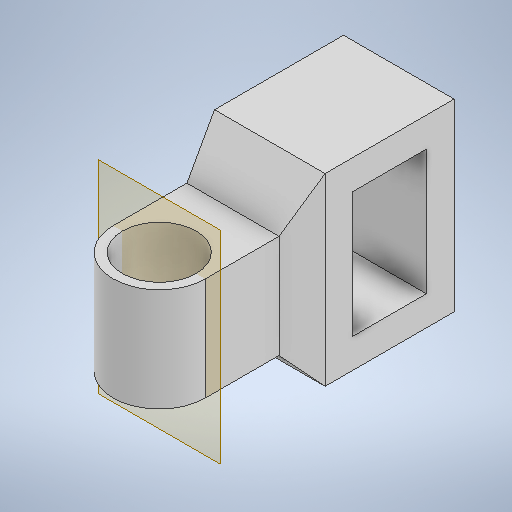
# Autodesk Inventor part: Part5
Saved by Autodesk Inventor 2025.2 (Build 292293000, 293)
## iProperties
Created: 2025-04-11
Part Number: Part5
Material: Generic
Document SubType Name: Sheet Metal
Designer: ziyuz
Density: 1 g/cm^3
Sheet Metal Rule: Default_mm
Appearance: Default
Author: ziyuz
Autodesk Inventor part; units mm, degrees
ref_plane "YZ Plane" through (0, 0, 0) normal (1, 0, 0) x (0, 1, 0)
ref_plane "XZ Plane" through (0, 0, 0) normal (0, 1, 0) x (-1, 0, 0)
sketch "Sketch1" plane through (0, 0, 0) normal (0, 1, 0) x (-1, 0, 0)
  circle A0 centre (0, 0) radius 10
  circle A1 centre (0, 0) radius 12.5
  dimension "d0" = 20
  dimension "d1" = 25
  constraints: 2 centre point, 2 coincident
  measures "d0" diameter of A0
  measures "d1" diameter of A1
extrude "Extrusion1" add sketch "Sketch1" along normal blind 28
sketch "Sketch2" plane through (0, 0, 0) normal (0, 0, 1) x (1, 0, 0)
  line L0 (12.5, 0) -> (-12.5, 0) projected
  line L1 (12.5, 28) -> (-12.5, 28) projected
  line L2 (-12.5, 0) -> (12.5, 0)
  line L3 (12.5, 0) -> (12.5, 28)
  line L4 (12.5, 28) -> (-12.5, 28)
  line L5 (-12.5, 28) -> (-12.5, 0)
  point P0 (0, 0)
  constraints: 8 end point, 2 parallel, 1 horizontal, 1 perpendicular
extrude "Extrusion2" add sketch "Sketch2" against normal blind 20
sketch "Sketch3" plane through (0, 28, 0) normal (0, 1, 0) x (1, 0, 0)
  circle A0 centre (0, 0) radius 10
  constraints: 1 centre point, 1 coincident
extrude "Extrusion3" cut sketch "Sketch3" against normal blind 50
ref_plane "Work Plane1" through (0, 0, -30) normal (0, 0, -1) x (-1, 0, 0)
sketch "Sketch4" plane through (0, 0, -30) normal (0, 0, -1) x (-1, 0, 0)
  line L0 (0, 0) -> (0, 28)
  line L1 (12.5, 28) -> (-12.5, 28) projected
  line L2 (-15, 30) -> (15, 30)
  line L3 (15, 30) -> (15, -2)
  line L4 (15, -2) -> (-15, -2)
  line L5 (-15, -2) -> (-15, 30)
  line L6 (-15, 30) -> (15, -2) construction
  line L7 (15, 30) -> (-15, -2) construction
  point P0 (0, 14)
  dimension "d9" = 30
  dimension "d10" = 32
  constraints: 14 end point, 4 midpoint, 2 parallel, 1 horizontal, 1 perpendicular
  measures "d9" distance of L3.end L4.end
  measures "d10" distance of L2.end L3.end
extrude "Extrusion4" add sketch "Sketch4" along normal blind 15
sketch "Sketch5" plane through (0, 0, -45) normal (0, 0, -1) x (-1, 0, 0)
  line L0 (15, 30) -> (-15, 30) projected
  line L1 (0, 30) -> (0, -2)
  line L2 (-15, -2) -> (15, -2) projected
  line L3 (-15, 39) -> (15, 39)
  line L4 (15, 39) -> (15, -11)
  line L5 (15, -11) -> (-15, -11)
  line L6 (-15, -11) -> (-15, 39)
  line L7 (-15, 39) -> (15, -11) construction
  line L8 (15, 39) -> (-15, -11) construction
  point P0 (0, 0)
  point P1 (0, 14)
  dimension "d17" = 30
  dimension "d18" = 50
  constraints: 14 end point, 5 midpoint, 2 parallel, 1 horizontal, 1 perpendicular
  measures "d17" distance of L4.end L5.end
  measures "d18" distance of L3.end L4.end
extrude "Extrusion5" add sketch "Sketch5" along normal blind 20 and the other way blind 15
sketch "Sketch7" plane through (15, -11, -30) normal (1, 0, 0) x (0, 0, -1)
  line L0 (0, 0) -> (35, 0) projected
  line L1 (17.5, 0) -> (17.5, 50)
  line L2 (35, 50) -> (0, 50) projected
  line L3 (35, 0) -> (35, 50) projected
  line L4 (35, 25) -> (0, 25)
  line L5 (0, 0) -> (0, 50) projected
  line L6 (7.5, 42) -> (27.5, 42)
  line L7 (27.5, 42) -> (27.5, 8)
  line L8 (27.5, 8) -> (7.5, 8)
  line L9 (7.5, 8) -> (7.5, 42)
  line L10 (7.5, 42) -> (27.5, 8) construction
  line L11 (27.5, 42) -> (7.5, 8) construction
  line L12 (27.5, 42) -> (7.5, 42)
  line L13 (7.5, 42) -> (7.5, 8)
  line L14 (7.5, 8) -> (27.5, 8)
  line L15 (27.5, 8) -> (27.5, 42)
  point P0 (-30, 11)
  point P1 (17.5, 25)
  dimension "d23" = 20
  dimension "d24" = 34
  constraints: 24 end point, 7 midpoint, 4 parallel, 2 horizontal, 2 perpendicular
  measures "d23" distance of L7.end L8.end
  measures "d24" distance of L6.end L7.end
extrude "Extrusion6" cut sketch "Sketch7" against normal blind 30 contours L8 L9 L4 L1 | L1 L4 L7 L8 | L9 L6 L1 L4 | L1 L6 L7 L4
loft "Loft2" add section 1 edges at (0, 28, -20) (12.5, 14, -20) (0, 0, -20) (-12.5, 14, -20) section 2 edges at (15, 14, -30) (0, 39, -30) (-15, 14, -30) (0, -11, -30)
equation "\"BendRadius\" = Thickness"
equation "\"BendReliefWidth\" = Thickness"
equation "\"BendReliefDepth\" = 0.5 * Thickness"
equation "\"CornerReliefSize\" = 4 * Thickness"
equation "\"MinimumRemnant\" = 2 * Thickness"
equation "\"TransitionRadius\" = BendRadius"
equation "\"JacobiRadiusSize\" = BendRadius"
equation "\"GapSize\" = Thickness"
equation "\"Thickness\" = 0.5"
body "Solid1"
